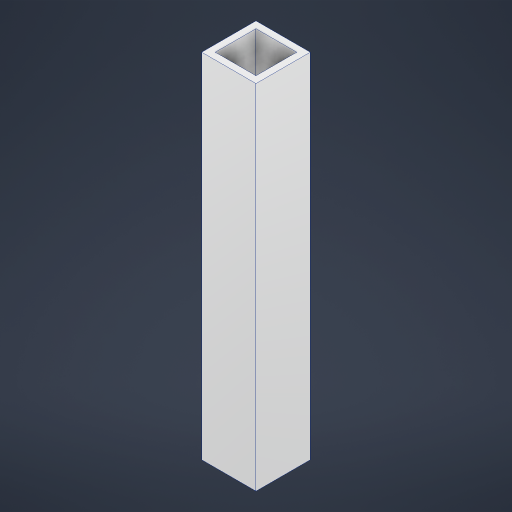
# Autodesk Inventor part: STRU_015_BilletPole_9in
Saved by Autodesk Inventor 2024.2 (Build 282272000, 272)
## iProperties
Created: 2024-07-25
Part Number: STRU_015_BilletPole_9in
Material: Aluminum 6061
Document SubType Name: Modeling
Designer: Bryan
Density: 2.7 g/cm^3
Appearance: Aluminum - Flat
Mass: 241.965 g
Surface Area: 570.16 cm^2
Volume: 89.6168 cm^3
Author: Bryan
Autodesk Inventor part; units mm, degrees
ref_plane "YZ Plane" through (0, 0, 0) normal (1, 0, 0) x (0, 1, 0)
ref_plane "XZ Plane" through (0, 0, 0) normal (0, 1, 0) x (-1, 0, 0)
ref_plane "XY Plane" through (0, 0, 0) normal (0, 0, 1) x (1, 0, 0)
sketch "Sketch1" plane through (0, 0, 0) normal (0, 1, 0) x (-1, 0, 0)
  line L0 (-12.7, -12.7) -> (12.7, -12.7)
  line L1 (12.7, -12.7) -> (12.7, 12.7)
  line L2 (12.7, 12.7) -> (-12.7, 12.7)
  line L3 (-12.7, 12.7) -> (-12.7, -12.7)
  line L4 (-12.7, -12.7) -> (12.7, 12.7) construction
  line L5 (12.7, -12.7) -> (-12.7, 12.7) construction
  line L6 (9.525, 9.525) -> (9.525, -9.525)
  line L7 (9.525, -9.525) -> (-9.525, -9.525)
  line L8 (-9.525, -9.525) -> (-9.525, 9.525)
  line L9 (-9.525, 9.525) -> (9.525, 9.525)
  point P0 (0, 0)
  dimension "d0" = 25.4
  dimension "d1" = 25.4
  dimension "d2" = 3.175
  constraints: 20 end point, 4 parallel, 2 midpoint, 2 perpendicular, 1 horizontal, 3 other
  measures "d0" distance of L2.end L1.end
  measures "d1" distance of L1.end L0.end
  measures "d2" distance between parallel lines of L1 L6
extrude "Extrusion1" add sketch "Sketch1" along normal blind 165.1
body "Solid1"
